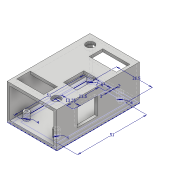
# Autodesk Inventor part: case_dcdc_concerter
Saved by Autodesk Inventor 2018 (Build 220112000, 112)
## iProperties
Created: 2017-11-21
Part Number: case_dcdc_concerter
Material: Generic
Document SubType Name: Modeling
Designer: Bardo91
Density: 1 g/cm^3
Appearance: Default
Author: Bardo91
Autodesk Inventor part; units mm, degrees
ref_plane "YZ Plane" through (0, 0, 0) normal (1, 0, 0) x (0, 1, 0)
ref_plane "XZ Plane" through (0, 0, 0) normal (0, 1, 0) x (-1, 0, 0)
ref_plane "XY Plane" through (0, 0, 0) normal (0, 0, 1) x (1, 0, 0)
sketch "Sketch1" plane through (0, 0, 0) normal (0, 0, 1) x (1, 0, 0)
  line L0 (0, 0) -> (26.5, 0)
  line L1 (26.5, 0) -> (26.5, 51)
  line L2 (26.5, 51) -> (0, 51)
  line L3 (0, 51) -> (0, 0)
  line L4 (-3, 54) -> (29.5, 54)
  line L5 (29.5, 54) -> (29.5, -3)
  line L6 (29.5, -3) -> (-3, -3)
  line L7 (-3, -3) -> (-3, 54)
  line L8 (31.5, 56) -> (-5, 56)
  line L9 (-5, 56) -> (-5, -5)
  line L10 (-5, -5) -> (31.5, -5)
  line L11 (31.5, -5) -> (31.5, 56)
  line L12 (-3, 54) -> (-3, 56)
  line L13 (29.5, 54) -> (29.5, 56)
  line L14 (29.5, -3) -> (29.5, -5)
  line L15 (-3, -3) -> (-3, -5)
  dimension "d0" = 26.5
  dimension "d1" = 51
  dimension "d2" = 3
  dimension "d3" = 2
  constraints: 32 end point, 6 parallel, 6 point on line, 5 perpendicular, 1 horizontal, 6 other
  measures "d0" distance of L2.end L1.end
  measures "d1" distance of L1.end L0.end
  measures "d2" distance between parallel lines of L2 L4
  measures "d3" distance between parallel lines of L4 L8
extrude "Extrusion1" add sketch "Sketch1" along normal blind 2 contours L3 L2 L1 L0 | L12 L8 L13 L4 | L4 L5 L6 L7 | L7 L15 L10 L9 L8 L12 | L13 L8 L11 L10 L14 L5 | L6 L14 L10 L15
extrude "Extrusion2" add sketch "Sketch1" along normal blind 24 contours L7 L15 L10 L9 L8 L12 | L13 L8 L11 L10 L14 L5
sketch "Sketch2" plane through (0, 0, 2) normal (0, 0, 1) x (1, 0, 0)
  line L0 (0, 0) -> (0, 51)
  line L1 (0, 25.5) -> (13.25, 25.5)
  line L2 (13.25, 25.5) -> (13.25, 49)
  line L3 (13.25, 49) -> (2.25, 49)
  circle A0 centre (2.25, 49) radius 1
  circle A1 centre (24.25, 49) radius 1
  circle A2 centre (2.25, 2) radius 1
  circle A3 centre (24.25, 2) radius 1
  circle A4 centre (2.25, 49) radius 2
  circle A5 centre (24.25, 49) radius 2
  circle A6 centre (2.25, 2) radius 2
  circle A7 centre (24.25, 2) radius 2
  dimension "d8" = 51
  dimension "d9" = 13.25
  dimension "d10" = 23.5
  dimension "d11" = 11
  dimension "d12" = 2
  dimension "d13" = 4
  dimension "d14" = 4
  dimension "d15" = 4
  dimension "d16" = 4
  constraints: 8 centre point, 8 end point, 5 coincident, 3 symmetric about line, 2 vertical, 1 horizontal, 1 midpoint, 1 perpendicular, 3 other
  measures "d8" distance of L0.start L0.end
  measures "d9" distance of L1.start L1.end
  measures "d10" distance of L1.end L2.end
  measures "d11" distance of L2.end L3.end
  measures "d12" diameter of A0
  measures "d13" diameter of A4
  measures "d14" diameter of A5
  measures "d15" diameter of A6
  measures "d16" diameter of A7
extrude "Extrusion3" add sketch "Sketch2" along normal blind 5
extrude "Extrusion4" cut sketch "Sketch2" against normal blind 5 contours A0 | A1 | A2 | A3
sketch "Sketch3" plane through (0, 0, 24) normal (0, 0, 1) x (1, 0, 0)
  line L0 (-5, 56) -> (-5, -5) projected
  line L1 (31.5, -5) -> (31.5, 56) projected
  line L2 (-5, -5) -> (31.5, -5)
  line L3 (31.5, -5) -> (31.5, 56)
  line L4 (31.5, 56) -> (-5, 56)
  line L5 (-5, 56) -> (-5, -5)
  point P0 (0, 0)
  constraints: 8 end point, 2 parallel, 1 horizontal, 1 perpendicular
extrude "Extrusion5" add sketch "Sketch3" along normal blind 2
sketch "Sketch4" plane through (0, 0, 26) normal (0, 0, 1) x (1, 0, 0)
  line L0 (29.5, -5) -> (29.5, 56) projected
  line L1 (29.5, 56) -> (29.5, 51)
  line L2 (29.5, 51) -> (9.5, 51)
  line L3 (9.5, 51) -> (9.5, 41)
  line L4 (9.5, 41) -> (29.5, 41)
  line L5 (29.5, 41) -> (29.5, 51)
  line L6 (-3, 56) -> (-3, -5) projected
  line L7 (-3, -5) -> (-3, 0)
  line L8 (-3, 0) -> (17, 0)
  line L9 (17, 0) -> (17, 10)
  line L10 (17, 10) -> (-3, 10)
  line L11 (-3, 10) -> (-3, 0)
  point P0 (0, 0)
  dimension "d23" = 5
  dimension "d24" = 20
  dimension "d25" = 10
  dimension "d26" = 20
  dimension "d27" = 5
  dimension "d28" = 20
  dimension "d29" = 10
  dimension "d30" = 20
  constraints: 20 end point, 4 perpendicular, 4 point on line
  measures "d23" distance of L0.end L1.end
  measures "d24" distance of L1.end L2.end
  measures "d25" distance of L2.end L3.end
  measures "d26" distance of L3.end L4.end
  measures "d27" distance of L6.end L7.end
  measures "d28" distance of L7.end L8.end
  measures "d29" distance of L8.end L9.end
  measures "d30" distance of L9.end L10.end
extrude "Extrusion6" cut sketch "Sketch4" against normal blind 2
sketch "Sketch5" plane through (0, 0, 26) normal (0, 0, 1) x (1, 0, 0)
  line L0 (-3, -5) -> (29.5, -5) projected
  line L1 (29.5, -5) -> (26.5, -5)
  line L2 (26.5, -5) -> (26.5, 15)
  line L3 (26.5, 15) -> (16.5, 15)
  line L4 (16.5, 15) -> (16.5, 30)
  line L5 (16.5, 30) -> (26.5, 30)
  line L6 (26.5, 30) -> (26.5, 15)
  circle A0 centre (24.25, 2) radius 2 projected
  circle A1 centre (24.25, 2) radius 3
  circle A2 centre (2.25, 49) radius 1 projected
  circle A3 centre (2.25, 49) radius 3
  point P0 (0, 0)
  dimension "d33" = 3
  dimension "d34" = 20
  dimension "d35" = 10
  dimension "d36" = 15
  dimension "d37" = 6
  dimension "d38" = 6
  constraints: 12 end point, 4 perpendicular, 2 centre point, 2 coincident, 1 point on line, 1 vertical
  measures "d33" distance of L0.end L1.end
  measures "d34" distance of L1.end L2.end
  measures "d35" distance of L2.end L3.end
  measures "d36" distance of L3.end L4.end
  measures "d37" diameter of A1
  measures "d38" diameter of A3
extrude "Extrusion7" cut sketch "Sketch5" against normal blind 2 contours A1 L2 | L3 L4 L5 L6 | L2 A1 | A0 | A2 | A3
sketch "Sketch6" plane through (31.5, -5, 0) normal (1, 0, 0) x (0, 0, -1)
  line L0 (-7, 5) -> (-7, 15)
  line L1 (-7, 15) -> (-20, 15)
  line L2 (-20, 15) -> (-20, 30)
  line L3 (-20, 30) -> (-7, 30)
  line L4 (-7, 30) -> (-7, 15)
  point P0 (0, 5)
  dimension "d41" = 10
  dimension "d42" = 13
  dimension "d43" = 15
  constraints: 10 end point, 3 perpendicular, 2 vertical
  measures "d41" distance of L0.start L0.end
  measures "d42" distance of L0.end L1.end
  measures "d43" distance of L1.end L2.end
extrude "Extrusion8" cut sketch "Sketch6" against normal blind 2
body "Solid1"
